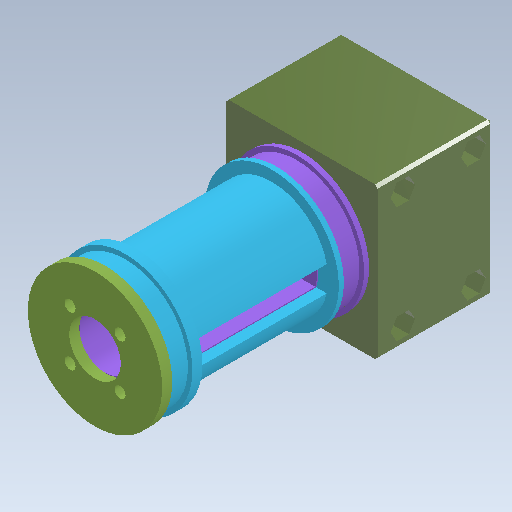
# Autodesk Inventor part: ForearmShaft2
Saved by Autodesk Inventor 2021 (Build 250183000, 183)
## iProperties
Created: 2020-02-16
Part Number: ForearmShaft2
Material: Generisch
Document SubType Name: Modeling
Designer: JochenAlt
Density: 1 g/cm^3
Appearance: Vorgabe
Author: JochenAlt
Autodesk Inventor part; units mm, degrees
note: some values were not read from the file. Left out: dimensions or parameters whose unit could not be read.
ref_plane "YZ Plane" through (0, 0, 0) normal (1, 0, 0) x (0, 1, 0)
ref_plane "XZ Plane" through (0, 0, 0) normal (0, 1, 0) x (-1, 0, 0)
sketch "Main" plane through (0, 0, 0) normal (0, 0, 1) x (1, 0, 0)
  line L0 (0, 37.6444) -> (0, -28.4407) construction
  line L1 (-34.1979, 0) -> (72.1871, 0) construction
  line L2 (0, -28.4407) -> (0, 37.6444) construction
  line L3 (-34.1979, 0) -> (72.1871, 0) construction
  circle A0 centre (0, 0) radius 19 construction
  arc A1 (-12.8789, -3.3204) -> (-9.6592, -9.1427) centre (0, 0) ccw
  circle A2 centre (0, 0) radius 13.3
  circle A3 centre (0, 0) radius 7 construction
  circle A4 centre (0, 0) radius 5.1
  circle A5 centre (-4.9497, -4.9497) radius 1.1
  circle A6 centre (4.9497, -4.9497) radius 1.1
  circle A7 centre (4.9497, 4.9497) radius 1.1
  circle A8 centre (-4.9497, 4.9497) radius 1.1
  circle A9 centre (0, 0) radius 9
  circle A10 centre (0, 0) radius 12.4
  circle A11 centre (0, 0) radius 9.2
  circle A12 centre (0, 0) radius 11.2
  line L4 (15, 15) -> (-15, 15)
  line L5 (-15, 15) -> (-15, -15)
  line L6 (-15, -15) -> (15, -15)
  line L7 (15, -15) -> (15, 15)
  line L8 (-4.9497, -4.9497) -> (4.9497, -4.9497) construction
  line L9 (4.9497, -4.9497) -> (4.9497, 4.9497) construction
  line L10 (-4.9497, 4.9497) -> (-4.9497, -4.9497) construction
  line L11 (-4.9497, 4.9497) -> (4.9497, 4.9497) construction
  line L12 (5.3282, 7.5) -> (-5.3282, 7.5)
  line L13 (5.3282, -7.5) -> (-5.3282, -7.5)
  point P0 (9.5, -16.4545)
  point P1 (9.5, 16.4545)
  point P2 (37.0107, 21.6054)
  point P3 (37.0107, 13.3946)
  point P4 (45.5607, 6.7963)
  point P5 (48.4393, 6.7963)
  point P6 (55.55, 10.9017)
  point P7 (56.9893, 13.3946)
  point P8 (56.9893, 21.6054)
  point P9 (55.55, 24.0983)
  point P10 (48.4393, 28.2037)
  point P11 (45.5607, 28.2037)
  point P12 (38.45, 24.0983)
  point P13 (-12.8789, -3.3204)
  point P14 (-4.1132, 5.664)
  point P15 (4.1132, 5.664)
  point P16 (5.664, 4.1132)
  point P17 (-4.1132, -5.664)
  point P18 (-5.664, -4.1132)
  point P19 (-5.664, 4.1132)
  point P20 (-4.9749, -7.5)
  point P21 (4.9749, -7.5)
  point P22 (4.9749, 7.5)
  point P23 (-4.9749, 7.5)
  dimension "d79" = 26.6
  dimension "d28" = 38
  dimension "d31" = 14
  dimension "d41" = 2.2
  dimension "d42" = 2
  dimension "d43" = 10.2
  dimension "d52" = 0.2
  dimension "d67" = 24.8
  dimension "d77" = 2
  dimension "d78" = 30
  dimension "d103" = 15
  constraints: 20 end point, 12 centre point, 12 point on circle, 11 coincident, 5 equal length, 3 equal radius, 3 horizontal, 3 parallel, 1 perpendicular, 5 other
  measures "d28" diameter of A0
  measures "d31" diameter of A3
  measures "d41" diameter of A5
  measures "d42" radial gap between concentric circles of A3 A9
  measures "d43" diameter of A4
  measures "d52" radial gap between concentric circles of A11 A9
  measures "d67" diameter of A10
  measures "d77" radial gap between concentric circles of A12 A11
  measures "d78" distance of L4.end L5.end
  measures "d103" distance between parallel lines of L13 L12
extrude "Extrusion21" add sketch "Main" along normal blind 22.8 contours A2 A1 | A9 L13 L12 | A9 L12 A11 L13 | L12 A9 | A9 L12 A11 | L13 A11 A9 | A9 L13 | A9 L13 A11 L12 | A10 | A12 | L7 L6 L5 L4
extrude "Extrusion22" cut sketch "Main" along normal blind 5 contours A5 | A6 | A7 | A8 | A9 L13 L12
extrude "Extrusion11" add sketch "Main" along normal blind 1 from surface at 22.8 separate body contours A2 A1 | A9 L13 L12 | A9 L12 A11 L13 | L12 A9 | A9 L12 A11 | L13 A11 A9 | A9 L13 | A9 L13 A11 L12 | A10 | A12
extrude "Extrusion13" add sketch "Main" along normal blind 4 from surface at 23.8 contours A9 L13 L12 | A9 L12 A11 L13 | L12 A9 | A9 L12 A11 | L13 A11 A9 | A9 L13 | A9 L13 A11 L12 | A10 | A12 bodies 2
extrude "Extrusion14" add sketch "Main" along normal blind 34 from surface at 27.8 contours A9 L13 L12 | L12 A9 | A9 L13 bodies 2
extrude "Extrusion15" add sketch "Main" along normal blind 30 from surface at 27.8 separate body contours A2 A1 | A10 | A12
extrude "Extrusion16" add sketch "Main" along normal blind 4 from surface at 57.8 contours A10 | A12 bodies 3
extrude "Extrusion17" add sketch "Main" along normal blind 2 from surface at 61.8 separate body contours A2 A1 | A9 L13 L12 | A9 L12 A11 L13 | L12 A9 | A9 L12 A11 | L13 A11 A9 | A9 L13 | A9 L13 A11 L12 | A10 | A12
ref_plane "Arbeitsebene3" through (0, 0, 55.8) normal (0, 0, 1) x (1, 0, 0)
sketch "Skizze3" plane through (0, 0, 55.8) normal (0, 0, -1) x (-1, 0, 0)
  circle A0 centre (0, 0) radius 5 construction
  line L0 (-13.0629, 2.5) -> (-4.3301, 2.5)
  line L1 (-4.3301, -2.5) -> (-13.0629, -2.5)
  line L2 (0, 0) -> (-13.3, 0) construction
  line L3 (0, 0) -> (13.3, 0) construction
  arc A1 (-4.3301, 2.5) -> (-4.3301, -2.5) centre (0, 0) ccw
  arc A2 (-13.0629, 2.5) -> (-13.0629, -2.5) centre (0, 0) ccw
  circle A3 centre (0, 0) radius 13.3 construction
  dimension "d62" = 180
  dimension "d63" = 5
  dimension "d93" = 10
  constraints: 8 end point, 7 point on circle, 4 coincident, 3 centre point, 1 collinear, 1 horizontal, 1 parallel, 3 other
  measures "d62" angle of L3 L2
  measures "d63" distance between parallel lines of L1 L0
  measures "d93" diameter of A0
extrude "Extrusion19" cut sketch "Skizze3" along normal blind 27 bodies 3 2
extrude "Extrusion20" cut sketch "Main" against normal up to surface (27 mm away) from surface at 55.8 contours A2 A1 | A10 bodies 3
sketch "Skizze4" plane through (0, 0, 0) normal (1, 0, 0) x (0, 1, 0)
  line L0 (-11.5, 17.8) -> (11.5, 17.8) construction
  line L1 (11.5, 17.8) -> (11.5, 3.8) construction
  line L2 (11.5, 3.8) -> (-11.5, 3.8) construction
  line L3 (-11.5, 3.8) -> (-11.5, 17.8) construction
  line L4 (0, -4.56) -> (0, 27.36) construction
  line L5 (-15, 0) -> (15, 0) construction
  circle A0 centre (-11.5, 17.8) radius 1.1
  circle A1 centre (-11.5, 3.8) radius 1.1
  circle A2 centre (11.5, 3.8) radius 1.1
  circle A3 centre (11.5, 17.8) radius 1.1
  circle A4 centre (11.5, 17.8) radius 2.1 construction
  circle A5 centre (11.5, 3.8) radius 2.1 construction
  circle A6 centre (-11.5, 17.8) radius 2.1 construction
  circle A7 centre (-11.5, 3.8) radius 2.1 construction
  line L6 (13.6, 16.5876) -> (11.5, 15.3751)
  line L7 (11.5, 15.3751) -> (9.4, 16.5876)
  line L8 (9.4, 16.5876) -> (9.4, 19.0124)
  line L9 (9.4, 19.0124) -> (11.5, 20.2249)
  line L10 (11.5, 20.2249) -> (13.6, 19.0124)
  line L11 (13.6, 19.0124) -> (13.6, 16.5876)
  line L12 (13.6, 2.5876) -> (11.5, 1.3751)
  line L13 (11.5, 1.3751) -> (9.4, 2.5876)
  line L14 (9.4, 2.5876) -> (9.4, 5.0124)
  line L15 (9.4, 5.0124) -> (11.5, 6.2249)
  line L16 (11.5, 6.2249) -> (13.6, 5.0124)
  line L17 (13.6, 5.0124) -> (13.6, 2.5876)
  line L18 (-9.4, 2.5876) -> (-11.5, 1.3751)
  line L19 (-11.5, 1.3751) -> (-13.6, 2.5876)
  line L20 (-13.6, 2.5876) -> (-13.6, 5.0124)
  line L21 (-13.6, 5.0124) -> (-11.5, 6.2249)
  line L22 (-11.5, 6.2249) -> (-9.4, 5.0124)
  line L23 (-9.4, 5.0124) -> (-9.4, 2.5876)
  line L24 (-9.4, 16.5876) -> (-11.5, 15.3751)
  line L25 (-11.5, 15.3751) -> (-13.6, 16.5876)
  line L26 (-13.6, 16.5876) -> (-13.6, 19.0124)
  line L27 (-13.6, 19.0124) -> (-11.5, 20.2249)
  line L28 (-11.5, 20.2249) -> (-9.4, 19.0124)
  line L29 (-9.4, 19.0124) -> (-9.4, 16.5876)
  point P0 (0, 0)
  point P1 (15, 22.8)
  point P2 (13.6, 17.8)
  point P3 (13.6, 3.8)
  point P4 (-9.4, 3.8)
  point P5 (-9.4, 17.8)
  dimension "d102" = 4.2
  dimension "d84" = 23
  dimension "d85" = 14
  dimension "d87" = 2.2
  dimension "d94" = 5
  constraints: 56 end point, 13 coincident, 4 centre point, 4 horizontal alignment, 4 midpoint, 4 point on line, 3 equal radius, 2 parallel, 1 horizontal, 1 perpendicular, 61 other
  measures "d84" distance of L1.end L2.end
  measures "d85" distance of L2.end L0.start
  measures "d87" diameter of A0
  measures "d94" distance from line of point (15, 22.8) L0
extrude "Extrusion23" cut sketch "Skizze4" along normal through all both and the other way through all contours A0 | A1 | A2 | A3 | L6 L7 L8 L9 L10 L11 | L12 L13 L14 L15 L16 L17 | L18 L19 L20 L21 L22 L23 | L24 L25 L26 L27 L28 L29 bodies 1
chamfer "Fase3" distance 0.5 angle 45 8 edges at (15, 15, 11.4) (-15, 15, 11.4) (15, -15, 11.4) (-15, -15, 11.4) (0, -15, 0) (0, 15, 0) (-15, 0, 0) (15, 0, 0)
sketch "Skizze5" plane through (0, 0, 0) normal (0, 0, -1) x (-1, 0, 0)
  arc A0 (-4.9749, 7.5) -> (-4.9749, -7.5) centre (0, 0) ccw construction
  line L0 (0, 4) -> (15, 4)
  line L1 (15, 4) -> (15, -4)
  line L2 (15, -4) -> (0, -4)
  line L3 (0, -4) -> (0, 4)
  line L4 (21, 0) -> (-21, 0) construction
  line L5 (0, -21) -> (0, 21) construction
  line L6 (15, -14.5) -> (15, 14.5) construction
  line L7 (15, 14.5) -> (15, -14.5) construction
  line L8 (15, 11.5) -> (15, 13.6) projected
  line L9 (15, 13.6) -> (15, 11.5) projected
  line L10 (15, 11.5) -> (15, 9.4) projected
  line L11 (15, 9.4) -> (15, 11.5) projected
  line L12 (15, -11.5) -> (15, -9.4) projected
  line L13 (15, -9.4) -> (15, -11.5) projected
  line L14 (15, -11.5) -> (15, -13.6) projected
  line L15 (15, -13.6) -> (15, -11.5) projected
  line L16 (4.9749, -7.5) -> (-4.9749, -7.5) projected
  line L17 (-4.9749, 7.5) -> (4.9749, 7.5) projected
  arc A1 (4.9749, -7.5) -> (4.9749, 7.5) centre (0, 0) ccw projected
  point P0 (15, -10.4)
  point P1 (15, -12.6)
  point P2 (15, 12.6)
  point P3 (15, 10.4)
  point P4 (15, -10.4)
  point P5 (15, -12.6)
  point P6 (15, 12.6)
  point P7 (15, 10.4)
  point P8 (15, 10.4)
  point P9 (15, -10.4)
  point P10 (15, -12.6)
  point P11 (15, 12.6)
  point P12 (15, 10.4)
  point P13 (15, -10.4)
  point P14 (15, -12.6)
  point P15 (15, 12.6)
  dimension "d98" = 8
  constraints: 8 end point, 2 perpendicular, 1 collinear, 1 horizontal, 1 point on line, 1 other
  measures "d98" distance of L0.end L1.end
extrude "Extrusion24" cut sketch "Skizze5" against normal blind 3 bodies 1
fillet "Rundung3" radius 2 1 edges at (-9, 0, 3)
equation "\"d52\" = tight_fit"
equation "\"roundness_small\" = 3"
equation "\"roundness_tiny\" = 0.5"
equation "\"wall_thickness\" = 3"
equation "\"medium_arm_width\" = 51"
equation "\"big_arm_width\" = 56"
equation "\"medium_arm_radius\" = 35"
equation "\"big_arm_radius\" = 48"
equation "\"medium_arm_circle_centre\" = 11"
equation "\"big_arm_circle_centre\" = 25"
equation "\"thickness\" = 3"
equation "\"tight_fit\" = 0.2"
equation "\"press_fit\" = 0.1"
equation "\"m2_hex_width\" = 4.2"
equation "\"m2_washer_diameter\" = 5.2"
equation "\"m2_screw_hole_diameter\" = 2.2"
equation "\"m2_allen_screw_width\" = 4"
equation "\"m2_allen_screw_height\" = 2"
equation "\"m2_washer_height\" = 0.3"
